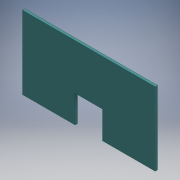
# Autodesk Inventor part: etage_support_minerai
Saved by Autodesk Inventor 2017 (Build 210142000, 142)
## iProperties
Created: 2017-04-16
Part Number: etage_support_minerai
Material: Generic
Document SubType Name: Modeling
Designer: franc
Density: 1 g/cm^3
Appearance: Default
Author: franc
Autodesk Inventor part; units mm, degrees
ref_plane "YZ Plane" through (0, 0, 0) normal (1, 0, 0) x (0, 1, 0)
ref_plane "XZ Plane" through (0, 0, 0) normal (0, 1, 0) x (-1, 0, 0)
ref_plane "XY Plane" through (0, 0, 0) normal (0, 0, 1) x (1, 0, 0)
sketch "Sketch1" plane through (0, 0, 0) normal (0, 1, 0) x (-1, 0, 0)
  line L0 (103.6486, 142.7027) -> (-186.3514, 142.7027)
  line L1 (-186.3514, 142.7027) -> (-186.3514, -17.2973)
  line L2 (103.6486, -17.2973) -> (103.6486, 142.7027)
  circle A0 centre (-41.3514, 138.2027) radius 1
  circle A1 centre (-41.3514, 122.2027) radius 1
  circle A2 centre (-33.3514, 130.2027) radius 1
  circle A3 centre (-49.3514, 130.2027) radius 1
  line L3 (-186.3514, -17.2973) -> (-71.3514, -17.2973)
  line L4 (-71.3514, -17.2973) -> (-71.3514, 42.7027)
  line L5 (-71.3514, 42.7027) -> (-11.3514, 42.7027)
  line L6 (-11.3514, 42.7027) -> (-11.3514, -17.2973)
  line L7 (-11.3514, -17.2973) -> (103.6486, -17.2973)
  point P0 (0, 0)
  dimension "d0" = 290
  dimension "d1" = 160
  dimension "d2" = 4.5
  dimension "d3" = 2
  dimension "d5" = 2
  dimension "d6" = 16
  dimension "d8" = 2
  dimension "d9" = 2
  dimension "d10" = 8
  dimension "d11" = 8
  dimension "d12" = 8
  dimension "d13" = 8
  dimension "d16" = 145
  dimension "d17" = 145
  dimension "d18" = 60
  dimension "d19" = 115
  dimension "d20" = 60
  constraints: 16 end point, 5 perpendicular, 4 centre point, 2 horizontal, 1 parallel, 1 point on line
  measures "d0" distance of L0.start L0.end
  measures "d1" distance of L2.start L0.start
  measures "d2" distance from line of L0 A0.centre
  measures "d3" diameter of A0
  measures "d5" diameter of A1
  measures "d6" distance of A1.centre A0.centre
  measures "d8" diameter of A2
  measures "d9" diameter of A3
  measures "d10" horizontal distance of A0.centre A2.centre
  measures "d11" horizontal distance of A3.centre A0.centre
  measures "d12" horizontal distance of A3.centre A0.centre
  measures "d13" horizontal distance of A2.centre A0.centre
  measures "d16" distance from line of L2 A1.centre
  measures "d17" distance from line of L2 A0.centre
  measures "d18" distance of L4.end L5.end
  measures "d19" distance of L1.end L3.end
  measures "d20" distance of L5.end L6.end
extrude "Extrusion1" add sketch "Sketch1" along normal blind 5
body "Solid1"
